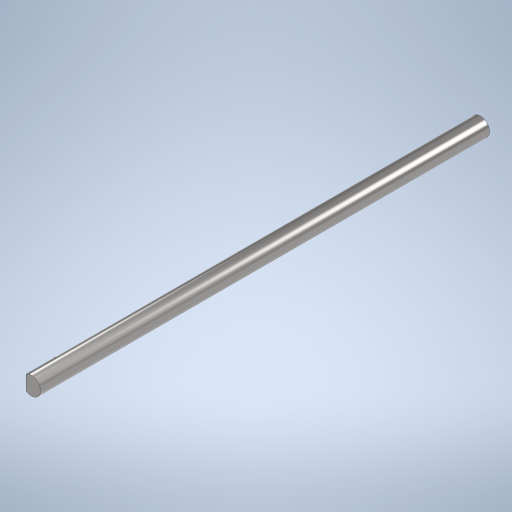
# Autodesk Inventor part: 12 mm rod
Saved by Autodesk Inventor 2023.2 (Build 272271000, 271)
## iProperties
Created: 2023-01-31
Part Number: 12 mm rod
Material: Steel, Mild
Document SubType Name: Modeling
Designer: dmargari
Density: 7.85 g/cm^3
Appearance: Semi-Polished
Author: dmargari
Autodesk Inventor part; units mm, degrees
ref_plane "YZ Plane" through (0, 0, 0) normal (1, 0, 0) x (0, 1, 0)
ref_plane "XZ Plane" through (0, 0, 0) normal (0, 1, 0) x (-1, 0, 0)
ref_plane "XY Plane" through (0, 0, 0) normal (0, 0, 1) x (1, 0, 0)
sketch "Sketch1" plane through (0, 0, 0) normal (0, 0, 1) x (1, 0, 0)
  circle A0 centre (0, 0) radius 6
  dimension "d0" = 12
  constraints: 1 centre point, 1 coincident
  measures "d0" diameter of A0
extrude "Extrusion1" add sketch "Sketch1" along normal mid plane 300
sketch "Sketch4" plane through (0, 0, 150) normal (0, 0, 1) x (1, 0, 0)
  circle A0 centre (0, 0) radius 6 projected
  line L0 (-3.652, -4.7606) -> (-3.652, 4.7606)
  constraints: 2 end point, 2 point on circle, 1 vertical
extrude "Extrusion4" cut sketch "Sketch4" against normal blind 20 contours L0 A0 picked at (-3.9806, -1.2689)
body "Solid1"
